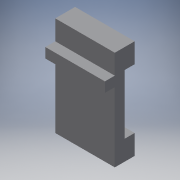
# Autodesk Inventor part: Slider
Saved by Autodesk Inventor 2016 (Build 200138000, 138)
## iProperties
Created: 2012-03-04
Part Number: Slider
Material: Generic
Document SubType Name: Modeling
Designer: John
Density: 1 g/cm^3
Appearance: Default
Author: John
Autodesk Inventor part; units mm, degrees
ref_plane "YZ Plane" through (0, 0, 0) normal (1, 0, 0) x (0, 1, 0)
ref_plane "XZ Plane" through (0, 0, 0) normal (0, 1, 0) x (-1, 0, 0)
ref_plane "XY Plane" through (0, 0, 0) normal (0, 0, 1) x (1, 0, 0)
sketch "Sketch1" plane through (0, 0, 0) normal (0, 0, 1) x (1, 0, 0)
  line L0 (0, 0) -> (76.2, 0)
  line L1 (76.2, 0) -> (76.2, 127)
  line L2 (76.2, 127) -> (0, 127)
  line L3 (0, 127) -> (0, 0)
  dimension "d0" = 76.2
  dimension "d1" = 127
  constraints: 8 end point, 2 parallel, 1 horizontal, 1 perpendicular
  measures "d0" distance of L2.end L1.end
  measures "d1" distance of L1.end L0.end
extrude "Extrusion1" add sketch "Sketch1" along normal blind 25.4
sketch "Sketch2" plane through (76.2, 0, 0) normal (1, 0, 0) x (0, 0, -1)
  line L0 (0, 0) -> (-25.4, 0) projected
  line L1 (0, 0) -> (0, 127) projected
  line L2 (0, 127) -> (-25.4, 127) projected
  line L3 (0, 25.4) -> (-12.7, 25.4)
  line L4 (-12.7, 25.4) -> (-12.7, 101.6)
  line L5 (-12.7, 101.6) -> (0, 101.6)
  line L6 (0, 101.6) -> (0, 25.4)
  dimension "d4" = 12.7
  dimension "d5" = 25.4
  dimension "d6" = 25.4
  constraints: 8 end point, 2 parallel, 1 horizontal, 1 perpendicular, 1 point on line
  measures "d4" distance of L4.end L5.end
  measures "d5" distance between parallel lines of L0 L3
  measures "d6" distance between parallel lines of L2 L5
extrude "Extrusion2" cut sketch "Sketch2" against normal through all
sketch "Sketch3" plane through (76.2, 0, 25.4) normal (1, 0, 0) x (0, 0, -1)
  line L0 (0, 127) -> (0, 0) projected
  line L1 (0, 88.9) -> (-12.7, 88.9)
  line L2 (-12.7, 88.9) -> (-12.7, 101.6)
  line L3 (-12.7, 101.6) -> (0, 101.6)
  line L4 (0, 101.6) -> (0, 88.9)
  line L5 (25.4, 127) -> (0, 127) projected
  dimension "d9" = 12.7
  dimension "d10" = 12.7
  dimension "d14" = 25.4
  constraints: 8 end point, 2 parallel, 1 horizontal, 1 perpendicular, 1 point on line
  measures "d9" distance of L1.end L2.end
  measures "d10" distance of L1.start L1.end
  measures "d14" distance between parallel lines of L5 L3
extrude "Extrusion3" add sketch "Sketch3" against normal up to surface (76.2 mm away) from surface at 0
equation "\"d6\" = d5"
body "Solid1"
